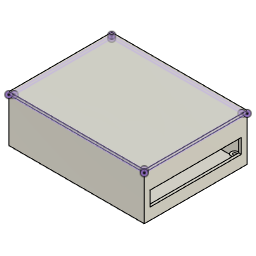
PCB Casing v2 (Autodesk Fusion 360 design; units mm, degrees)
Autodesk Fusion 360 part; units mm, degrees
sketch "Base" plane through (0, 0, 0) normal (0, 0, 1) x (1, 0, 0)
  line L0 (41.6, 31.6) -> (-41.6, 31.6)
  line L1 (-41.6, 31.6) -> (-41.6, -31.6)
  line L2 (-41.6, -31.6) -> (41.6, -31.6)
  line L3 (41.6, -31.6) -> (41.6, 31.6)
  line L4 (41.6, 31.6) -> (-41.6, -31.6) construction
  line L5 (-41.6, 31.6) -> (41.6, -31.6) construction
  point P0 (-41.6, 0)
  dimension "d1" = 83.2
  dimension "d2" = 63.2
  constraint horizontal L0
  constraint perpendicular L0 L1
  constraint parallel L0 L2
  constraint parallel L1 L3
  constraint coincident L4 origin
  constraint coincident L5 origin
  constraint midpoint L1 P0
  measures "d1" distance of L1.end L2.end
  measures "d2" distance of L0.end L1.end
extrude "Extrusion1" add sketch "Base" along normal blind 28.7 makes body 1
shell "Schale1" thickness 1.6 removed faces 0 bodies 1
ref_plane "Arbeitsebene1" through (-40, -30, 1.6) normal (0, 0, -1) x (-1, 0, 0)
sketch "Skizze3" plane through (-27.6, -16.7, 1.6) normal (0, 0, -1) x (1, 0, 0)
  line L0 (-12.4, 13.3) -> (67.6, 13.3)
  line L1 (-12.4, -46.7) -> (-12.4, 13.3)
  circle A0 centre (-10.15, 11.05) radius 2.25
  line L2 (67.6, -46.7) -> (-12.4, -46.7)
  circle A1 centre (-10.15, -44.45) radius 2.25
  line L3 (67.6, 13.3) -> (67.6, -46.7)
  circle A2 centre (65.35, -44.45) radius 2.25
  circle A3 centre (65.35, 11.05) radius 2.25
  circle A4 centre (-10.15, 11.05) radius 0.9
  circle A5 centre (-10.15, -44.45) radius 0.9
  circle A6 centre (65.35, -44.45) radius 0.9
  circle A7 centre (65.35, 11.05) radius 0.9
  dimension "d7" = 2.25
  dimension "d8" = 2.25
  dimension "d9" = 2.25
  dimension "d10" = 2.25
  dimension "d19" = 1.8
  dimension "d20" = 1.8
  dimension "d21" = 1.8
  dimension "d22" = 1.8
  constraint tangent L0 A0
  constraint tangent L1 A0
  constraint tangent L2 A1
  constraint tangent L1 A1
  constraint tangent L2 A2
  constraint tangent L3 A2
  constraint tangent L3 A3
  constraint tangent L0 A3
  constraint concentric A0 A4
  constraint concentric A1 A5
  constraint concentric A2 A6
  constraint concentric A3 A7
  measures "d7" radius of A0
  measures "d8" radius of A1
  measures "d9" radius of A2
  measures "d10" radius of A3
  measures "d19" diameter of A4
  measures "d20" diameter of A5
  measures "d21" diameter of A6
  measures "d22" diameter of A7
extrude "Extrusion2" add sketch "Skizze3" against normal blind 4 contours A0 | A3 | A1 | A2 bodies 1
ref_plane "Arbeitsebene2" through (0, 0, 27.1) normal (0, 0, 1) x (1, 0, 0)
split "Teilen1" by plane through (0, 0, 27.1) normal (0, 0, 1) bodies 1 makes body 2 at (-13.8667, 10.5333, 28.7)
sketch "Skizze6" plane through (0, 0, 27.1) normal (0, 0, 1) x (1, 0, 0)
  line L0 (40, -30) -> (-40, -30)
  line L1 (-40, -30) -> (-40, 30)
  line L2 (-40, 30) -> (40, 30)
  line L3 (40, 30) -> (40, -30)
  line L4 (-41.6, -31.6) -> (41.6, -31.6)
  line L5 (41.6, -31.6) -> (41.6, 31.6)
  line L6 (41.6, 31.6) -> (-41.6, 31.6)
  line L7 (-41.6, 31.6) -> (-41.6, -31.6)
sketch "Skizze7" plane through (0, 0, 27.1) normal (0, 0, 1) x (1, 0, 0)
  line L0 (40, -30) -> (-40, -30)
  line L1 (-40, -30) -> (-40, 30)
  line L2 (-40, 30) -> (40, 30)
  line L3 (40, 30) -> (40, -30)
  line L4 (-41.6, -31.6) -> (41.6, -31.6)
  line L5 (41.6, -31.6) -> (41.6, 31.6)
  line L6 (41.6, 31.6) -> (-41.6, 31.6)
  line L7 (-41.6, 31.6) -> (-41.6, -31.6)
  line L8 (-39.9, 29.9) -> (39.9, 29.9)
  line L9 (39.9, 29.9) -> (39.9, -29.9)
  line L10 (39.9, -29.9) -> (-39.9, -29.9)
  line L11 (-39.9, -29.9) -> (-39.9, 29.9)
  line L12 (-39, 29) -> (39, 29)
  line L13 (39, 29) -> (39, -29)
  line L14 (39, -29) -> (-39, -29)
  line L15 (-39, -29) -> (-39, 29)
  point P0 (-40, -30)
  dimension "d34" = 0.1
  dimension "d35" = 1
extrude "Extrusion5" add sketch "Skizze7" against normal blind 1 contours L8 L9 L10 L11 bodies 2
sketch "Hole" plane through (-41.6, 0, 0) normal (-1, 0, 0) x (0, -1, 0)
  line L0 (-31.6, 0) -> (31.6, 0)
  line L1 (31.6, 0) -> (31.6, 27.1)
  line L2 (31.6, 28.7) -> (-31.6, 28.7)
  line L3 (-31.6, 27.1) -> (-31.6, 0)
  line L4 (-28, 16.1) -> (28, 16.1)
  line L5 (28, 16.1) -> (28, 7.1)
  line L6 (28, 7.1) -> (-28, 7.1)
  line L7 (-28, 7.1) -> (-28, 16.1)
  line L8 (27.75, 1.6) -> (30, 1.6)
  line L9 (-27.75, 1.6) -> (27.75, 1.6)
  line L10 (-30, 1.6) -> (-27.75, 1.6)
  line L11 (31.6, 27.1) -> (-31.6, 27.1)
  line L12 (-31.6, 27.1) -> (31.6, 27.1)
  line L13 (31.6, 27.1) -> (31.6, 28.7)
  line L14 (-31.6, 28.7) -> (-31.6, 27.1)
  point P0 (0, 7.1)
  dimension "d13" = 56
  dimension "d14" = 9
  dimension "d40" = 7.1
  constraint horizontal L4
  constraint vertical L5
  constraint horizontal L6
  constraint vertical L7
  constraint midpoint L6 P0
  constraint vertical origin P0
  measures "d13" distance of L4.start L4.end
  measures "d14" distance of L4.start L6.end
  measures "d40" distance of L0 L6
extrude "Extrusion3" cut sketch "Hole" against normal blind 83.2 contours L4 L5 L6 L7 bodies 1
equation "d1 = pcb_length + 2 * wall_thickness"
equation "d2 = pcb_width + 2 * wall_thickness"
equation "d3 = case_internal_height + 2 * wall_thickness"
equation "d5 = wall_thickness"
equation "wall_thickness = 1.6 mm"
equation "d7 = socket_width / 2"
equation "d8 = socket_width / 2"
equation "d9 = socket_width / 2"
equation "d10 = socket_width / 2"
equation "d11 = -pcb_space_below"
equation "d13 = pcb_width - ( 2 * 2 ) * 1 mm"
equation "d14 = hole_height"
equation "d17 = -2 * wall_thickness - pcb_length"
equation "d19 = socket_hole_with"
equation "d20 = socket_hole_with"
equation "d21 = socket_hole_with"
equation "d22 = socket_hole_with"
equation "d23 = -wall_thickness"
equation "pcb_width = 60 mm"
equation "pcb_length = 80 mm"
equation "case_internal_height = pcb_space_above + pcb_space_below + pcb_thickness" comment "max. 33mm in front, 40mm in back side"
equation "pcb_space_below = 4 mm"
equation "pcb_thickness = 1.5 mm"
equation "pcb_space_above = 20 mm"
equation "socket_hole_with = 1.8 mm"
equation "socket_width = 4.5 mm" comment "measured from walls"
equation "d40 = wall_thickness + pcb_space_below + pcb_thickness"
equation "hole_height = 9 mm" comment "for usb and cables"
named bodies: "Case lower", "Case upper"
